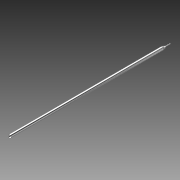
# Autodesk Inventor part: pipette
Saved by Autodesk Inventor 2011 SP2 (Build 150309200, 309)
## iProperties
Created: 2013-09-16
Part Number: pipette
Document SubType Name: Modeling
Designer: sungwook
Density: 1 g/cm^3
Author: sungwook
Autodesk Inventor part; units mm, degrees
ref_plane "YZ Plane" through (0, 0, 0) normal (1, 0, 0) x (0, 1, 0)
ref_plane "XZ Plane" through (0, 0, 0) normal (0, 1, 0) x (-1, 0, 0)
ref_plane "XY Plane" through (0, 0, 0) normal (0, 0, 1) x (1, 0, 0)
sketch "Sketch1" plane through (0, 0, 0) normal (0, 0, 1) x (1, 0, 0)
  circle A0 centre (0, 0) radius 0.5207
  dimension "d0" = 1.0414
  constraints: 1 centre point, 1 coincident
  measures "d0" diameter of A0
sketch "Sketch1 outline for Extrusion1" plane through (0, 0, 0) normal (0, 0, 1) x (1, 0, 0)
  circle A0 centre (0, 0) radius 0.5207
extrude "Extrusion1" add sketch "Sketch1 outline for Extrusion1" along normal blind 53.5432
sketch "Sketch3" plane through (0, 0, 0) normal (0, 1, 0) x (-1, 0, 0)
  line L0 (0, -10.70864) -> (0, 64.25184)
  line L1 (-0.5207, 0) -> (0.5207, 0)
  line L2 (-0.5207, 0) -> (-0.5207, 53.5432)
  line L3 (0.5207, 0) -> (0.5207, 53.5432)
  line L4 (0.4572, 0) -> (0.4572, 53.5432)
  line L5 (-0.5207, 53.5432) -> (0.5207, 53.5432)
  line L6 (0.0508, 0) -> (0, 0)
  line L7 (0, 0) -> (0, 3)
  line L8 (0, 3) -> (0.0508, 3)
  line L9 (0.0508, 3) -> (0.0508, 0)
  line L10 (0, 0) -> (0.1143, 0)
  line L11 (0.1143, 0) -> (0.1143, 3)
  line L12 (0.1143, 3) -> (0, 3)
  line L13 (0, 3) -> (0, 0)
  line L14 (0, 3) -> (0.5207, 3)
  spline S0 degree 4 poles (0.1143, 0) (0.1143, 0.51605) (0.092329, 2.145399) (0.396023, 1.739504) (0.5207, 2.685768) (0.5207, 3) knots 0 0 0 0 0 0.53463216 1 1 1 1 1
  spline S1 degree 4 poles (0.0508, 0) (0.0508, 0.513555) (0.032096, 2.101955) (0.338843, 1.754797) (0.4572, 2.685063) (0.4572, 3) knots 0 0 0 0 0 0.53394472 1 1 1 1 1
  line L15 (0, 54.462693) -> (0.4572, 54.462693)
  line L16 (0.4572, 54.462693) -> (0.4572, 3)
  line L17 (0.4572, 3) -> (0, 3)
  line L18 (0, 3) -> (0, 54.462693)
  point P0 (0.390046, 2.157892)
  point P1 (0.22686, 1.754843)
  point P2 (0.164132, 1.732429)
  point P3 (0.330809, 2.160123)
  point P4 (0.2286, 54.462693)
  dimension "d7" = 3
  dimension "d8" = 0.0508
  dimension "d17" = 0.0635
  dimension "d18" = 0.0635
  constraints: 28 end point, 7 parallel, 7 point on line, 4 perpendicular, 4 vertical, 3 horizontal, 1 midpoint, 9 other
  measures "d7" distance between parallel lines of L8 L6
  measures "d8" distance between parallel lines of L0 L9
  measures "d17" distance between parallel lines of L4 L3
  measures "d18" distance between parallel lines of L9 L11
sketch "Sketch3 outline for Revolution1" plane through (0, 0, 0) normal (0, 1, 0) x (-1, 0, 0)
  spline S0 degree 4 poles (0.1143, 0) (0.1143, 0.51605) (0.092329, 2.145399) (0.396023, 1.739504) (0.5207, 2.685768) (0.5207, 3) knots 0 0 0 0 0 0.53463216 1 1 1 1 1
  line L0 (0.5207, 0) -> (0.5207, 3)
  line L1 (0.4572, 0) -> (0.5207, 0)
  line L2 (0.1143, 0) -> (0.4572, 0)
revolve "Revolution1" cut sketch "Sketch3 outline for Revolution1" angle 360 about axis through (0, 0, -10) along (0, 0, 1)
sketch "Sketch3 outline for Revolution2" plane through (0, 0, 0) normal (0, 1, 0) x (-1, 0, 0)
  line L0 (0, 0) -> (0.0508, 0)
  line L1 (0.0508, 0) -> (0.0508, 0.358012)
  spline S0 degree 4 poles (0.0508, 0.358012) (0.052632, 0.873182) (0.082062, 2.052843) (0.348737, 1.832558) (0.4572, 2.685063) (0.4572, 3) knots 0 0 0 0 0 0.49143364 1 1 1 1 1
  line L2 (0.4572, 3) -> (0, 3)
  line L3 (0, 3) -> (0, 0)
revolve "Revolution2" cut sketch "Sketch3 outline for Revolution2" angle 360 about axis through (0, 0, -10) along (0, 0, 1)
sketch "Sketch3 outline for Revolution3" plane through (0, 0, 0) normal (0, 1, 0) x (-1, 0, 0)
  line L0 (0, 3) -> (0.4572, 3)
  line L1 (0, 54.462693) -> (0, 3)
  line L2 (0.4572, 54.462693) -> (0, 54.462693)
  line L3 (0.4572, 3) -> (0.4572, 54.462693)
revolve "Revolution3" cut sketch "Sketch3 outline for Revolution3" angle 360 about axis through (0, 0, -10) along (0, 0, 1)
body "Solid1"
